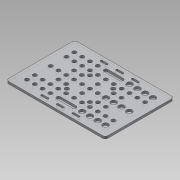
# Autodesk Inventor part: V-Slot Universal Build Plate
Saved by Autodesk Inventor 2016 (Build 200138000, 138)
## iProperties
Created: 2013-06-19
Part Number: V-Slot Universal Build Plate
Material: Aluminum 6061
Document SubType Name: Modeling
Designer: Jon Hollander
Density: 2.71 g/cm^3
Appearance: Aluminum - Flat
Author: Jon Hollander
Autodesk Inventor part; units mm, degrees
ref_plane "YZ Plane" through (0, 0, 0) normal (1, 0, 0) x (0, 1, 0)
ref_plane "XZ Plane" through (0, 0, 0) normal (0, 1, 0) x (-1, 0, 0)
sketch "Sketch1" plane through (0, 0, 0) normal (0, 0, 1) x (1, 0, 0)
  line L0 (0, 0) -> (127, 0)
  line L1 (127, 0) -> (127, 88)
  line L2 (127, 88) -> (0, 88)
  line L3 (0, 88) -> (0, 0)
  dimension "d0" = 127
  dimension "d1" = 88
  constraints: 8 end point, 2 parallel, 1 horizontal, 1 perpendicular
  measures "d0" distance of L2.end L1.end
  measures "d1" distance of L1.end L0.end
extrude "Extrusion1" add sketch "Sketch1" along normal blind 3
fillet "Fillet1" radius 3.36 4 edges at (0, 88, 1.5) (0, 0, 1.5) (127, 0, 1.5) (127, 88, 1.5)
sketch "Sketch4" plane through (0, 0, 3) normal (0, 0, 1) x (1, 0, 0)
  line L0 (123.64, 88) -> (3.36, 88) projected
  line L1 (0, 84.64) -> (0, 3.36) projected
  line L2 (3.36, 0) -> (123.64, 0) projected
  line L3 (127, 3.36) -> (127, 84.64) projected
  line L4 (0, 74.32) -> (127, 74.32) construction
  line L5 (0, 64.32) -> (127, 64.32) construction
  line L6 (0, 44) -> (127, 44) construction
  line L7 (0, 23.68) -> (127, 23.68) construction
  line L8 (0, 13.68) -> (127, 13.68) construction
  line L9 (63.5, 88) -> (63.5, 0) construction
  point P0 (0, 0)
  point P1 (63.5, 64.32)
  point P2 (53.34, 64.32)
  point P3 (43.18, 64.32)
  point P4 (33.18, 64.32)
  point P5 (23.18, 64.32)
  point P6 (13.18, 64.32)
  point P7 (73.66, 64.32)
  point P8 (83.82, 64.32)
  point P9 (93.82, 64.32)
  point P10 (103.82, 64.32)
  point P11 (113.82, 64.32)
  point P12 (63.5, 23.68)
  point P13 (53.34, 23.68)
  point P14 (43.18, 23.68)
  point P15 (33.18, 23.68)
  point P16 (23.18, 23.68)
  point P17 (13.18, 23.68)
  point P18 (113.82, 23.68)
  point P19 (103.82, 23.68)
  point P20 (93.82, 23.68)
  point P21 (83.82, 23.68)
  point P22 (73.66, 23.68)
  point P23 (63.5, 44)
  point P24 (43.18, 44)
  point P25 (33.18, 44)
  point P26 (23.18, 44)
  point P27 (13.18, 44)
  point P28 (53.5, 44)
  point P29 (73.5, 44)
  point P30 (43.18, 74.32)
  point P31 (33.18, 74.32)
  point P32 (23.18, 74.32)
  point P33 (13.18, 74.32)
  point P34 (43.18, 13.68)
  point P35 (33.18, 13.68)
  point P36 (23.18, 13.68)
  point P37 (13.18, 13.68)
  dimension "d37" = 13.68
  dimension "d38" = 23.68
  dimension "d39" = 44
  dimension "d40" = 64.32
  dimension "d41" = 74.32
  dimension "d42" = 10.16
  dimension "d43" = 20.32
  dimension "d46" = 10
  dimension "d55" = 10.16
  dimension "d56" = 20.32
  dimension "d57" = 10
  dimension "d62" = 20.32
  dimension "d63" = 10
  dimension "d64" = 10
  constraints: 20 point on line, 12 end point, 6 midpoint, 6 symmetric about line, 4 perpendicular, 1 horizontal, 3 other
  measures "d37" distance between parallel lines of L4 L0
  measures "d38" distance between parallel lines of L5 L0
  measures "d39" distance between parallel lines of L0 L6
  measures "d40" distance between parallel lines of L0 L7
  measures "d41" distance between parallel lines of L8 L0
  measures "d42" distance of point (63.5, 64.32) point (53.34, 64.32)
  measures "d43" distance of point (63.5, 64.32) point (43.18, 64.32)
  measures "d46" distance of point (43.18, 64.32) point (33.18, 64.32)
  measures "d55" distance of point (63.5, 23.68) point (53.34, 23.68)
  measures "d56" distance of point (63.5, 23.68) point (43.18, 23.68)
  measures "d57" distance of point (43.18, 23.68) point (33.18, 23.68)
  measures "d62" distance of point (63.5, 44) point (43.18, 44)
  measures "d63" distance of point (43.18, 44) point (33.18, 44)
  measures "d64" distance of point (63.5, 44) point (53.5, 44)
hole "Hole2" at (63.5, 64.32, 3) at (53.34, 64.32, 3) at (43.18, 64.32, 3) at (33.18, 64.32, 3) at (23.18, 64.32, 3) at (13.18, 64.32, 3) at (113.82, 64.32, 3) at (103.82, 64.32, 3) at (93.82, 64.32, 3) at (83.82, 64.32, 3) at (73.66, 64.32, 3) at (73.66, 23.68, 3) at (83.82, 23.68, 3) at (93.82, 23.68, 3) at (103.82, 23.68, 3) at (113.82, 23.68, 3) at (13.18, 23.68, 3) at (23.18, 23.68, 3) at (33.18, 23.68, 3) at (43.18, 23.68, 3) at (53.34, 23.68, 3) at (63.5, 23.68, 3) at (13.18, 44, 3) at (23.18, 44, 3) at (33.18, 44, 3) at (43.18, 44, 3) at (63.5, 44, 3) at (53.5, 44, 3) at (73.5, 44, 3) at (43.18, 74.32, 3) at (33.18, 74.32, 3) at (23.18, 74.32, 3) at (13.18, 74.32, 3) at (43.18, 13.68, 3) at (33.18, 13.68, 3) at (23.18, 13.68, 3) at (13.18, 13.68, 3) direction (0, 0, -1) diameter 5 end through all
sketch "Sketch5" plane through (0, 0, 3) normal (0, 0, 1) x (1, 0, 0)
  circle A0 centre (13.18, 44) radius 2.5 projected
  circle A1 centre (13.18, 74.32) radius 2.5 projected
  circle A2 centre (13.18, 13.68) radius 2.5 projected
  line L0 (123.64, 88) -> (3.36, 88) projected
  line L1 (3.36, 0) -> (123.64, 0) projected
  line L2 (127, 3.36) -> (127, 84.64) projected
  line L3 (13.18, 74.32) -> (127, 74.32) construction
  line L4 (13.18, 44) -> (127, 44) construction
  line L5 (13.18, 13.68) -> (127, 13.68) construction
  line L6 (63.5, 88) -> (63.5, 0) construction
  point P0 (0, 0)
  point P1 (83.82, 74.32)
  point P2 (93.82, 74.32)
  point P3 (103.82, 74.32)
  point P4 (113.82, 74.32)
  point P5 (83.82, 44)
  point P6 (93.82, 44)
  point P7 (103.82, 44)
  point P8 (113.82, 44)
  point P9 (83.82, 13.68)
  point P10 (93.82, 13.68)
  point P11 (103.82, 13.68)
  point P12 (113.82, 13.68)
  constraints: 14 point on line, 8 end point, 3 midpoint, 2 perpendicular
hole "Hole3" at (83.82, 74.32, 3) at (93.82, 74.32, 3) at (103.82, 74.32, 3) at (113.82, 74.32, 3) at (83.82, 44, 3) at (93.82, 44, 3) at (103.82, 44, 3) at (113.82, 44, 3) at (83.82, 13.68, 3) at (93.82, 13.68, 3) at (103.82, 13.68, 3) at (113.82, 13.68, 3) direction (0, 0, -1) diameter 7.14 end through all
sketch "Sketch6" plane through (0, 0, 3) normal (0, 0, 1) x (1, 0, 0)
  line L0 (123.64, 88) -> (3.36, 88) projected
  line L1 (0, 84.64) -> (0, 3.36) projected
  line L2 (3.36, 0) -> (123.64, 0) projected
  line L3 (127, 3.36) -> (127, 84.64) projected
  line L4 (0, 5.98) -> (127, 5.98) construction
  line L5 (63.5, 88) -> (63.5, 0) construction
  line L6 (66.99, 4.73) -> (60.01, 4.73)
  line L7 (60.01, 7.23) -> (66.99, 7.23)
  line L8 (66.99, 4.73) -> (60.01, 7.23) construction
  line L9 (60.01, 4.73) -> (66.99, 7.23) construction
  arc A0 (60.01, 7.23) -> (60.01, 4.73) centre (59.9902, 5.98) ccw
  arc A1 (66.99, 4.73) -> (66.99, 7.23) centre (66.99, 5.98) ccw
  line L10 (86.99, 4.73) -> (80.01, 4.73)
  line L11 (80.01, 7.23) -> (86.99, 7.23)
  line L12 (86.99, 4.73) -> (80.01, 7.23) construction
  line L13 (80.01, 4.73) -> (86.99, 7.23) construction
  arc A2 (80.01, 7.23) -> (80.01, 4.73) centre (79.9902, 5.98) ccw
  arc A3 (86.99, 4.73) -> (86.99, 7.23) centre (86.99, 5.98) ccw
  line L14 (46.99, 4.73) -> (40.01, 4.73)
  line L15 (40.01, 7.23) -> (46.99, 7.23)
  line L16 (46.99, 4.73) -> (40.01, 7.23) construction
  line L17 (40.01, 4.73) -> (46.99, 7.23) construction
  arc A4 (40.01, 7.23) -> (40.01, 4.73) centre (39.9902, 5.98) ccw
  arc A5 (46.99, 4.73) -> (46.99, 7.23) centre (46.99, 5.98) ccw
  line L18 (66.99, 4.73) -> (60.01, 4.73)
  line L19 (60.01, 7.23) -> (66.99, 7.23)
  line L20 (66.99, 4.73) -> (60.01, 7.23) construction
  line L21 (60.01, 4.73) -> (66.99, 7.23) construction
  arc A6 (60.01, 7.23) -> (60.01, 4.73) centre (59.9902, 5.98) ccw
  arc A7 (66.99, 4.73) -> (66.99, 7.23) centre (66.99, 5.98) ccw
  line L22 (0, 44) -> (127, 44) construction
  point P0 (0, 0)
  point P1 (63.5, 5.98)
  point P2 (83.5, 5.98)
  point P3 (43.5, 5.98)
  point P4 (63.5, 5.98)
  dimension "d79" = 5.98
  dimension "d82" = 6.98
  dimension "d83" = 2.5
  dimension "d84" = 9.5
  dimension "d87" = 20
  dimension "d90" = 20
  constraints: 38 end point, 16 point on circle, 13 midpoint, 8 centre point, 4 point on line, 3 horizontal, 2 tangent, 1 parallel, 1 perpendicular, 39 other
  measures "d79" distance between parallel lines of L2 L4
  measures "d82" distance of L7.end L7.start
  measures "d83" distance between parallel lines of L6 L7
  measures "d87" distance of A0.centre A2.centre
  measures "d90" distance of A0.centre A4.centre
extrude "Extrusion2" cut sketch "Sketch6" against normal up to next
ref_plane "Work Plane1" through (3.36, 44, 0) normal (0, -1, 0) x (1, 0, 0)
mirror "Mirror1" about plane through (3.36, 44, 0) normal (0, -1, 0) of "Extrusion2"
sketch "Sketch7" plane through (0, 0, 3) normal (0, 0, 1) x (1, 0, 0)
  line L0 (86.99, 80.77) -> (80.01, 80.77) projected
  line L1 (80.01, 83.27) -> (86.99, 83.27) projected
  circle A0 centre (13.18, 13.68) radius 2.5 projected
  line L2 (123.64, 88) -> (3.36, 88) projected
  line L3 (3.36, 0) -> (123.64, 0) projected
  line L4 (127, 3.36) -> (127, 84.64) projected
  line L5 (13.18, 13.68) -> (127, 13.68) construction
  line L6 (63.5, 88) -> (63.5, 0) construction
  line L7 (53.5, 16.18) -> (73.5, 16.18)
  line L8 (73.5, 11.18) -> (53.5, 11.18)
  line L9 (51, 16.18) -> (76, 11.18) construction
  line L10 (76, 16.18) -> (51, 11.18) construction
  arc A1 (53.5, 16.18) -> (53.5, 11.18) centre (53.5, 13.68) ccw
  arc A2 (73.5, 11.18) -> (73.5, 16.18) centre (73.5, 13.68) ccw
  point P0 (0, 0)
  point P1 (63.5, 13.68)
  dimension "d95" = 25
  dimension "d96" = 13.68
  dimension "d97" = 20
  dimension "d98" = 2.5
  dimension "d99" = 2.5
  dimension "d100" = 11.31
  dimension "d101" = 11.31
  dimension "d102" = 51
  dimension "d103" = 51
  dimension "d104" = 53.5
  dimension "d105" = 76
  constraints: 12 end point, 5 tangent, 4 midpoint, 4 point on circle, 3 point on line, 2 centre point, 1 horizontal, 1 parallel, 1 perpendicular
  measures "d95" distance of L9.end L10.end
  measures "d96" distance from line of L3 point (63.5, 13.68)
  measures "d97" distance of A2.centre A1.centre
  measures "d98" radius of A1
  measures "d99" radius of A2
  measures "d100" angle of L0 L9
  measures "d101" angle of L1 L10
  measures "d102" distance from line of L10.start L4
  measures "d103" distance from line of L9.end L4
  measures "d104" distance from line of L7.end L4
  measures "d105" distance from line of L9.start L4
extrude "Extrusion3" cut sketch "Sketch7" against normal up to next contours L7 A2 L8 A1
mirror "Mirror2" about plane through (3.36, 44, 0) normal (0, -1, 0) of "Extrusion3"
sketch "Sketch8" plane through (0, 0, 3) normal (0, 0, 1) x (1, 0, 0)
  circle A0 centre (43.18, 44) radius 2.5 projected
  line L0 (123.64, 88) -> (3.36, 88) projected
  line L1 (0, 84.64) -> (0, 3.36) projected
  line L2 (3.36, 0) -> (123.64, 0) projected
  line L3 (127, 3.36) -> (127, 84.64) projected
  line L4 (63.5, 88) -> (63.5, 0) construction
  line L5 (0, 44) -> (127, 44) construction
  line L6 (63.5, 34) -> (0, 34) construction
  point P0 (0, 0)
  point P1 (63.5, 54)
  point P2 (43.18, 34)
  point P3 (33.18, 34)
  point P4 (83.82, 34)
  point P5 (93.82, 34)
  point P6 (43.18, 54)
  point P7 (33.18, 54)
  point P8 (93.82, 54)
  point P9 (83.82, 54)
  dimension "d108" = 34
  dimension "d109" = 10
  constraints: 7 symmetric about line, 6 end point, 4 midpoint, 4 point on line, 1 perpendicular, 1 vertical alignment
  measures "d108" distance from line of L2 L6.start
  measures "d109" distance of point (43.18, 34) point (33.18, 34)
hole "Hole4" at (63.5, 34, 3) at (63.5, 54, 3) at (43.18, 34, 3) at (33.18, 34, 3) at (93.82, 34, 3) at (83.82, 34, 3) at (33.18, 54, 3) at (43.18, 54, 3) at (83.82, 54, 3) at (93.82, 54, 3) direction (0, 0, -1) diameter 5 end through all
sketch "Sketch9" plane through (0, 0, 3) normal (0, 0, 1) x (1, 0, 0)
  circle A0 centre (63.5, 44) radius 2.5 projected
  line L0 (123.64, 88) -> (3.36, 88) projected
  line L1 (0, 84.64) -> (0, 3.36) projected
  line L2 (3.36, 0) -> (123.64, 0) projected
  line L3 (127, 3.36) -> (127, 84.64) projected
  line L4 (0, 44) -> (127, 44) construction
  line L5 (63.5, 88) -> (63.5, 0) construction
  line L6 (78.325, 88) -> (78.325, 0) construction
  line L7 (0, 58.82) -> (127, 58.82) construction
  point P0 (0, 0)
  point P1 (78.325, 58.82)
  point P2 (78.325, 29.18)
  point P3 (48.675, 58.82)
  point P4 (48.675, 29.18)
  dimension "d117" = 14.82
  dimension "d118" = 14.825
  constraints: 8 end point, 6 point on line, 4 midpoint, 3 symmetric about line, 2 perpendicular
  measures "d117" distance from line of A0.centre L7
  measures "d118" distance from line of L6 A0.centre
hole "Hole5" at (78.325, 58.82, 3) at (78.325, 29.18, 3) at (48.675, 58.82, 3) at (48.675, 29.18, 3) direction (0, 0, -1) diameter 5 end through all
body "Solid1"
